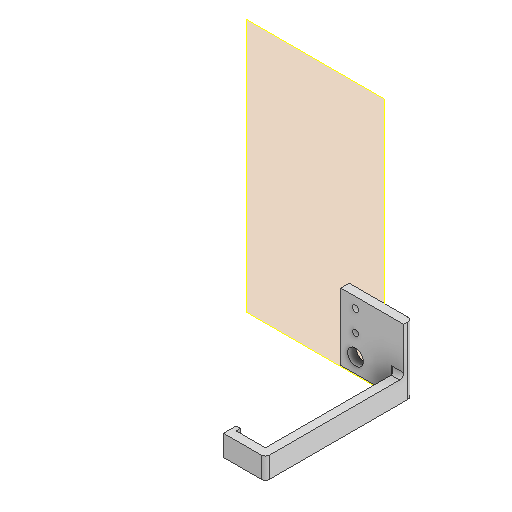
# Autodesk Inventor part: 30_XY_Sample_lightsheetarm_sample_v3
Saved by Autodesk Inventor 2022 (Build 260153000, 153)
## iProperties
Created: 2021-11-10
Part Number: 30_XY_Sample_lightsheetarm_sample_v3
Material: Generic
Document SubType Name: Modeling
Designer: diederichbenedict
Density: 1 g/cm^3
Appearance: Default
Author: diederichbenedict
Autodesk Inventor part; units mm, degrees
ref_plane "YZ Plane" through (0, 0, 0) normal (1, 0, 0) x (0, 1, 0)
ref_plane "XZ Plane" through (0, 0, 0) normal (0, 1, 0) x (-1, 0, 0)
ref_plane "XY Plane" through (0, 0, 0) normal (0, 0, 1) x (1, 0, 0)
ref_plane "Work Plane1" through (0, 0, 0) normal (0, 0, 1) x (1, 0, 0)
sketch "Sketch1" plane through (0, 0, 0) normal (0, 0, 1) x (1, 0, 0)
  line L0 (-30, -73.2876) -> (-18.6416, -61.9292) projected
  line L1 (-18.6416, -61.9292) -> (-17.5809, -62.9898) projected
  line L2 (-17.5809, -62.9898) -> (-30, -75.4089) projected
  line L3 (-30, -75.4089) -> (-30, -76) projected
  arc A0 (-30, -76) -> (-26, -80) centre (-26, -76) ccw projected
  line L4 (-18, -80) -> (-26, -80) projected
  arc A1 (-18, -80) -> (-14, -76) centre (-18, -76) ccw projected
  line L5 (-14, -34) -> (-14, -76) projected
  arc A2 (-10, -30) -> (-14, -34) centre (-10, -34) ccw projected
  line L6 (-10, -30) -> (12, -30) projected
  arc A3 (16, -34) -> (12, -30) centre (12, -34) ccw projected
  line L7 (16, -34) -> (16, -76) projected
  arc A4 (16, -76) -> (20, -80) centre (20, -76) ccw projected
  line L8 (20, -80) -> (26, -80) projected
  arc A5 (26, -80) -> (30, -76) centre (26, -76) ccw projected
  line L9 (30, 28) -> (30, -76) projected
  line L10 (30, 28) -> (28, 30) projected
  line L11 (28, 30) -> (-28, 30) projected
  line L12 (-28, 30) -> (-30, 28) projected
  line L13 (-30, 28) -> (-30, -73.2876) projected
  circle A6 centre (-10, -25) radius 1.45 projected
  circle A7 centre (-10, 25) radius 1.45 projected
  circle A8 centre (10, 25) radius 1.45 projected
  circle A9 centre (10, -25) radius 1.45 projected
  circle A10 centre (25, -10) radius 1.45 projected
  circle A11 centre (-25, -10) radius 1.45 projected
  circle A12 centre (-25, 10) radius 1.45 projected
  circle A13 centre (25, 10) radius 1.45 projected
  circle A14 centre (-17.5, -17.5) radius 1.95 projected
  circle A15 centre (17.5, 17.5) radius 1.95 projected
  circle A16 centre (17.5, -17.5) radius 1.95 projected
  circle A17 centre (-17.5, 17.5) radius 1.95 projected
  circle A18 centre (-25, 25) radius 2.325 projected
  circle A19 centre (25, -25) radius 2.325 projected
  circle A20 centre (-25, -25) radius 2.325 projected
  circle A21 centre (25, 25) radius 2.325 projected
  circle A22 centre (0, 0) radius 16 projected
  circle A23 centre (23, -74) radius 3.75 projected
  circle A24 centre (23, -64) radius 1.45 projected
  circle A25 centre (23, -54) radius 1.45 projected
  line L14 (16, -49) -> (46, -49)
  line L15 (46, -49) -> (46, -81)
  line L16 (46, -81) -> (16, -81)
  line L17 (16, -81) -> (16, -49)
  point P0 (0, 0)
  dimension "d0" = 30
  dimension "d1" = 32
  dimension "d2" = 5
  constraints: 8 end point, 2 parallel, 1 horizontal, 1 perpendicular, 1 point on line
  measures "d0" distance of L15.end L16.end
  measures "d1" distance of L14.end L15.end
  measures "d2" distance from line of L14 A25.centre
extrude "Extrusion1" add sketch "Sketch1" along normal blind 4 contours L14 L15 L16 L17 A4 L8 A5 L9 | L9 A5 L8 A4 L7 L14
sketch "Sketch2" plane through (16, -81, 0) normal (0, -1, 0) x (1, 0, 0)
  line L0 (0, 0) -> (30, 0) projected
  line L1 (30, 0) -> (30, 4) projected
  line L2 (0, 4) -> (30, 4) projected
  line L3 (0, 0) -> (0, 4) projected
  line L4 (30, 4) -> (26, 4)
  line L5 (26, 4) -> (26, 66)
  line L6 (26, 66) -> (30, 66)
  line L7 (30, 66) -> (30, 4)
  line L8 (30, 66) -> (10, 66)
  line L9 (10, 66) -> (10, 70)
  line L10 (10, 70) -> (30, 70)
  line L11 (30, 70) -> (30, 66)
  point P0 (-16, 0)
  point P1 (26, 4)
  dimension "d5" = 4
  dimension "d6" = 62
  dimension "d7" = 20
  dimension "d8" = 4
  constraints: 16 end point, 4 parallel, 2 horizontal, 2 perpendicular
  measures "d5" distance of L5.end L6.end
  measures "d6" distance of L4.end L5.end
  measures "d7" distance of L9.end L10.end
  measures "d8" distance of L8.end L9.end
extrude "Extrusion2" add sketch "Sketch2" against normal blind 10 contours L2 L5 L6 L7 | L6 L8 L9 L10 L11
fillet "Fillet1" radius 2 4 edges at (46, -76, 70) (42, -76, 4) (44, -71, 4) (46, -65, 0)
sketch "Sketch3" plane through (16, -81, 0) normal (0, -1, 0) x (1, 0, 0)
  line L0 (10, 66) -> (10, 70) projected
  line L1 (10, 66) -> (12, 66)
  line L2 (12, 66) -> (12, 64)
  line L3 (12, 64) -> (10, 64)
  line L4 (10, 64) -> (10, 66)
  point P0 (-16, 0)
  dimension "d12" = 2
  dimension "d13" = 2
  constraints: 8 end point, 2 parallel, 1 horizontal, 1 perpendicular
  measures "d12" distance of L2.end L3.end
  measures "d13" distance of L1.end L2.end
extrude "Extrusion3" add sketch "Sketch3" against normal blind 10
body "Solid1"
